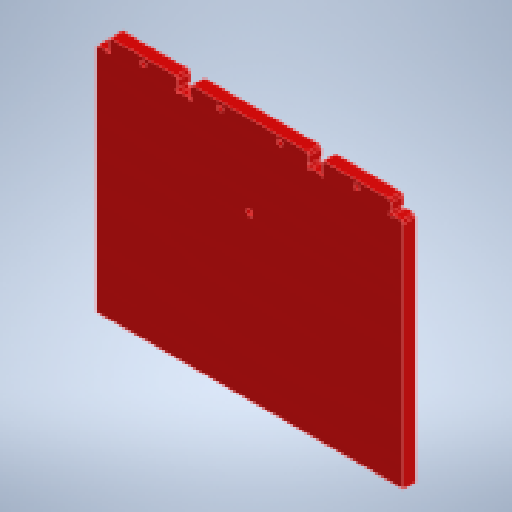
# Autodesk Inventor part: 부품49
Saved by Autodesk Inventor 2024 (Build 280153000, 153)
## iProperties
Created: 2024-09-07
Part Number: 부품49
Material: PMMA 플라스틱
Document SubType Name: Modeling
Designer: Eungang
Density: 1.188 g/cm^3
Appearance: 빨간색
Mass: 82.7023 g
Surface Area: 268.811 cm^2
Volume: 69.6147 cm^3
Author: Eungang
Autodesk Inventor part; units mm, degrees
ref_plane "YZ Plane" through (0, 0, 0) normal (1, 0, 0) x (0, 1, 0)
ref_plane "XZ Plane" through (0, 0, 0) normal (0, 1, 0) x (-1, 0, 0)
ref_plane "XY Plane" through (0, 0, 0) normal (0, 0, 1) x (1, 0, 0)
sketch "스케치1" plane through (0, 0, 0) normal (0, 0, 1) x (1, 0, 0)
  line L0 (118.1968, 6) -> (118.1968, 0)
  line L1 (0, 0) -> (2.3, 0) projected
  line L2 (2.3, 0) -> (2.3, -6) projected
  line L3 (150, -6) -> (2.3, -6) projected
  line L4 (150, -6) -> (150, 6) projected
  line L5 (0, 6) -> (150, 6) projected
  line L6 (0, 0) -> (0, 6) projected
  line L7 (150, -6) -> (0, -6)
  line L8 (0, -6) -> (0, 0)
  line L9 (0, 0) -> (150, 0)
  line L10 (150, 0) -> (150, -6)
  line L11 (150, -6) -> (144, -6)
  line L12 (144, -6) -> (144, 0)
  line L13 (144, 0) -> (150, 0)
  line L14 (150, 0) -> (150, -6)
  line L15 (122.25, 6) -> (131.75, 6) projected
  line L16 (128.025, 6) -> (128.025, 0)
  line L17 (125.975, 6) -> (125.975, 0)
  line L18 (127, 0) -> (127, 6)
  line L19 (104, 0) -> (104, -6)
  line L20 (104, -6) -> (110, -6)
  line L21 (110, -6) -> (110, 0)
  line L22 (110, 0) -> (104, 0)
  line L23 (104, 0) -> (104, -6)
  line L24 (75, -6) -> (75, 6)
  line L25 (0, 0) -> (0, -6)
  line L26 (0, -6) -> (6, -6)
  line L27 (6, 0) -> (0, 0)
  line L28 (0, 0) -> (0, -6)
  line L29 (40, 0) -> (46, 0)
  line L30 (150, -6) -> (144, -6)
  line L31 (144, -6) -> (144, 0)
  line L32 (144, 0) -> (150, 0)
  line L33 (150, 0) -> (150, -6)
  line L34 (110, -6) -> (104, -6)
  line L35 (104, -6) -> (104, 0)
  line L36 (104, 0) -> (110, 0)
  line L37 (110, 0) -> (110, -6)
  line L38 (0, 0) -> (0, -6)
  line L39 (0, -6) -> (6, -6)
  line L40 (6, -6) -> (6, 0)
  line L41 (6, 0) -> (0, 0)
  line L42 (0, 0) -> (0, -6)
  line L43 (40, -6) -> (40, 0)
  line L44 (46, -6) -> (40, -6)
  line L45 (46, 0) -> (46, -6)
  line L46 (46, 0) -> (46, -6)
  line L47 (40, 0) -> (46, 0)
  line L48 (0, -6) -> (6, -6)
  line L49 (6, -6) -> (6, 0)
  line L50 (6, 0) -> (0, 0)
  line L51 (0, 0) -> (0, -6)
  line L52 (40, -6) -> (46, -6)
  line L53 (46, -6) -> (46, 0)
  line L54 (46, 0) -> (40, 0)
  line L55 (40, 0) -> (40, -6)
  line L56 (150, 0) -> (0, 0)
  line L57 (0, 0) -> (0, -125.2)
  line L58 (0, -125.2) -> (150, -125.2)
  line L59 (150, -125.2) -> (150, 0)
  line L60 (150, -62.6) -> (0, -62.6)
  line L61 (0, -125.2) -> (2.3, -125.2)
  line L62 (2.3, -125.2) -> (2.3, -119.2)
  line L63 (150, -119.2) -> (2.3, -119.2)
  line L64 (150, -119.2) -> (0, -119.2)
  line L65 (0, -119.2) -> (0, -125.2)
  line L66 (0, -125.2) -> (150, -125.2)
  line L67 (150, -125.2) -> (150, -119.2)
  line L68 (150, -119.2) -> (144, -119.2)
  line L69 (144, -119.2) -> (144, -125.2)
  line L70 (144, -125.2) -> (150, -125.2)
  line L71 (150, -125.2) -> (150, -119.2)
  line L72 (110, -119.2) -> (110, -125.2)
  line L73 (104, -119.2) -> (110, -119.2)
  line L74 (104, -125.2) -> (104, -119.2)
  line L75 (104, -125.2) -> (104, -119.2)
  line L76 (110, -125.2) -> (104, -125.2)
  line L77 (40, -125.2) -> (46, -125.2)
  line L78 (0, -125.2) -> (0, -119.2)
  line L79 (0, -119.2) -> (6, -119.2)
  line L80 (0, -125.2) -> (0, -119.2)
  line L81 (6, -125.2) -> (0, -125.2)
  line L82 (150, -119.2) -> (144, -119.2)
  line L83 (144, -119.2) -> (144, -125.2)
  line L84 (144, -125.2) -> (150, -125.2)
  line L85 (150, -125.2) -> (150, -119.2)
  line L86 (110, -119.2) -> (104, -119.2)
  line L87 (104, -119.2) -> (104, -125.2)
  line L88 (104, -125.2) -> (110, -125.2)
  line L89 (110, -125.2) -> (110, -119.2)
  line L90 (0, -125.2) -> (0, -119.2)
  line L91 (0, -119.2) -> (6, -119.2)
  line L92 (6, -119.2) -> (6, -125.2)
  line L93 (6, -125.2) -> (0, -125.2)
  line L94 (0, -125.2) -> (0, -119.2)
  line L95 (6, -119.2) -> (6, -125.2)
  line L96 (0, -125.2) -> (0, -119.2)
  line L97 (0, -119.2) -> (6, -119.2)
  line L98 (6, -125.2) -> (0, -125.2)
  line L99 (40, -119.2) -> (40, -125.2)
  line L100 (40, -125.2) -> (40, -119.2)
  line L101 (46, -119.2) -> (40, -119.2)
  line L102 (46, -125.2) -> (46, -119.2)
  line L103 (46, -125.2) -> (46, -119.2)
  line L104 (46, -119.2) -> (46, -125.2)
  line L105 (40, -119.2) -> (46, -119.2)
  line L106 (46, -125.2) -> (40, -125.2)
  line L107 (40, -125.2) -> (46, -125.2)
  line L108 (150, -125.2) -> (0, -125.2)
  point P0 (21.975, 0)
  point P1 (24.025, 0)
  point P2 (31.8032, 0)
  point P3 (21.975, 0)
  point P4 (24.025, 0)
  point P5 (23, 0)
  point P6 (118.1968, -125.2)
  point P7 (128.025, -125.2)
  point P8 (125.975, -125.2)
  point P9 (127, -125.2)
  point P10 (75, -119.2)
  point P11 (24.025, -125.2)
  point P12 (21.975, -125.2)
  point P13 (24.025, -125.2)
  point P14 (23, -125.2)
  point P15 (21.975, -125.2)
  point P16 (31.8032, -125.2)
  dimension "d0" = 125.2
  constraints: 204 end point, 79 symmetric about line, 10 parallel, 5 horizontal, 5 midpoint, 5 perpendicular, 4 point on line, 3 vertical, 6 other
  measures "d0" distance of L57.end L56.end
extrude "돌출1" add sketch "스케치1" along normal blind 6 contours L9 L12 L3 L21 | L24 L3 L45 L9 | L9 L19 L3 L24 | L3 L59 L60 L57 L7 | L43 L3 L40 L9 | L60 L59 L63 L64 L57
sketch "스케치2" plane through (0, 0, 0) normal (0, 0, -1) x (-1, 0, 0)
  circle A0 centre (-72.2193, -29.1573) radius 1.55 projected
  circle A1 centre (-75, -39.8) radius 1.5 projected
  circle A2 centre (-75, -39.8) radius 13.9 projected
  circle A3 centre (-75, -39.8) radius 5.2 projected
  circle A4 centre (-75, -39.8) radius 1.6
  point P0 (0, 0)
  dimension "d5" = 0.1
  constraints: 1 centre point
  measures "d5" radial gap between concentric circles of A1 A4
extrude "돌출2" cut sketch "스케치2" against normal up to next contours A1 | A4
sketch "스케치5" plane through (0, 0, 6) normal (0, 0, 1) x (1, 0, 0)
  line L0 (6, 0) -> (6, -6) projected
  line L1 (6, -6) -> (0, -6) projected
  line L2 (0, -6) -> (0, -119.2) projected
  line L3 (150, -119.2) -> (150, -6) projected
  line L4 (150, -6) -> (144, -6) projected
  line L5 (144, -6) -> (144, 0) projected
  line L6 (144, 0) -> (110, 0) projected
  line L7 (110, 0) -> (110, -6) projected
  line L8 (110, -6) -> (104, -6) projected
  line L9 (104, -6) -> (104, 0) projected
  line L10 (104, 0) -> (46, 0) projected
  line L11 (46, 0) -> (46, -6) projected
  line L12 (46, -6) -> (40, -6) projected
  line L13 (40, -6) -> (40, 0) projected
  line L14 (40, 0) -> (6, 0) projected
  circle A0 centre (75, -39.8) radius 1.6 projected
  circle A1 centre (40, -6) radius 1
  circle A2 centre (46, -6) radius 1
  circle A3 centre (40, 0) radius 1
  circle A4 centre (46, 0) radius 1
  circle A5 centre (6, 0) radius 1
  line L15 (6, 0) -> (6, -6) projected
  circle A6 centre (6, -6) radius 1
  circle A7 centre (0, -6) radius 1
  circle A8 centre (104, -6) radius 1
  circle A9 centre (104, 0) radius 1
  line L16 (110, -6) -> (104, -6) projected
  circle A10 centre (110, -6) radius 1
  circle A11 centre (110, 0) radius 1
  circle A12 centre (144, -6) radius 1
  line L17 (144, 0) -> (110, 0) projected
  circle A13 centre (144, 0) radius 1
  circle A14 centre (150, -6) radius 1
  circle A15 centre (123.8, -69.5) radius 1
  circle A16 centre (123.8, -63.1) radius 1
  circle A17 centre (130.2, -69.5) radius 1
  line L18 (130.2, -69.5) -> (130.2, -63.1) projected
  circle A18 centre (130.2, -63.1) radius 1
  circle A19 centre (19.8, -69.5) radius 1
  circle A20 centre (19.8, -63.1) radius 1
  circle A21 centre (26.2, -69.5) radius 1
  circle A22 centre (26.2, -63.1) radius 1
  line L19 (0, -119.2) -> (150, -119.2) projected
  point P0 (0, 0)
  point P1 (149, -6)
  point P2 (150, -7)
  point P3 (144, -5)
  point P4 (145, -6)
  point P5 (143, 0)
  point P6 (144, -1)
  dimension "d32" = 2
  dimension "d33" = 2
  dimension "d34" = 2
  dimension "d35" = 2
  dimension "d36" = 2
  dimension "d37" = 2
  dimension "d38" = 2
  dimension "d39" = 2
  dimension "d40" = 2
  dimension "d41" = 2
  dimension "d42" = 2
  dimension "d43" = 2
  dimension "d44" = 2
  dimension "d45" = 2
  dimension "d46" = 2
  dimension "d47" = 2
  dimension "d48" = 2
  dimension "d49" = 2
  dimension "d50" = 2
  dimension "d51" = 2
  dimension "d52" = 2
  dimension "d53" = 2
  constraints: 22 centre point, 16 coincident
  measures "d32" diameter of A1
  measures "d33" diameter of A2
  measures "d34" diameter of A3
  measures "d35" diameter of A4
  measures "d36" diameter of A5
  measures "d37" diameter of A6
  measures "d38" diameter of A7
  measures "d39" diameter of A8
  measures "d40" diameter of A9
  measures "d41" diameter of A10
  measures "d42" diameter of A11
  measures "d43" diameter of A12
  measures "d44" diameter of A13
  measures "d45" diameter of A14
  measures "d46" diameter of A15
  measures "d47" diameter of A16
  measures "d48" diameter of A17
  measures "d49" diameter of A18
  measures "d50" diameter of A19
  measures "d51" diameter of A20
  measures "d52" diameter of A21
  measures "d53" diameter of A22
extrude "돌출5" cut sketch "스케치5" against normal up to next contours L14 A5 L0 | L0 A5 L14 | A6 L1 L0 | L0 L1 A6 | A3 L13 L14 | L14 L13 A3 | A7 L2 L1 | L1 L2 A7 | A1 L12 L13 | L13 L12 A1 | A2 L11 L12 | L12 L11 A2 | A14 L4 L3 | A4 L10 L11 | L11 L10 A4 | A12 L5 L4 | A9 L9 L10 | L10 L9 A9 | A13 L6 L5 | A8 L8 L9 | L9 L8 A8 | A11 L7 L6 | L6 L7 A11 | A10 L7 L8 | L8 L7 A10 picked at (149.7812, -6.6253) picked at (143.8112, -6.634) picked at (143.7812, -0.6253)
sketch "스케치6" plane through (0, 0, 6) normal (0, 0, 1) x (1, 0, 0)
  line L0 (6, -6) -> (6, 0) projected
  line L1 (0, 0) -> (6, 0) projected
  line L2 (0, -6) -> (0, 0) projected
  line L3 (0, -6) -> (6, -6) projected
  line L4 (40, 0) -> (40, -6) projected
  line L5 (40, -6) -> (46, -6) projected
  line L6 (46, -6) -> (46, 0) projected
  line L7 (40, 0) -> (46, 0) projected
  line L8 (40, 0) -> (6, 0)
  line L9 (23, 0) -> (23, -6)
  circle A0 centre (23, -3) radius 1.35
  line L10 (104, 0) -> (104, -6) projected
  line L11 (104, -6) -> (110, -6) projected
  line L12 (110, -6) -> (110, 0) projected
  line L13 (104, 0) -> (110, 0) projected
  line L14 (144, 0) -> (144, -6) projected
  line L15 (144, -6) -> (150, -6) projected
  line L16 (150, -6) -> (150, 0) projected
  line L17 (144, 0) -> (150, 0) projected
  line L18 (104, -3) -> (46, -3)
  line L19 (75, -3) -> (75, 0)
  line L20 (103, 0) -> (47, 0) projected
  line L21 (75, -3) -> (104, -3)
  line L22 (89.5, -3) -> (89.5, 0)
  line L23 (75, -3) -> (46, -3)
  line L24 (60.5, -3) -> (60.5, 0)
  circle A1 centre (89.5, -3) radius 1.3
  circle A2 centre (60.5, -3) radius 1.3
  circle A3 centre (127, -3) radius 1.35
  point P0 (127, -6)
  dimension "d58" = 2.6
  dimension "d59" = 2.6
  constraints: 16 end point, 8 midpoint, 4 centre point, 2 coincident, 2 collinear, 2 perpendicular, 2 symmetric about line, 2 vertical, 1 point on line, 1 other
  measures "d58" diameter of A1
  measures "d59" diameter of A2
extrude "돌출6" cut sketch "스케치6" against normal up to next contours A0 L9 | L9 A0 | A1 L18 | L18 L22 A1 | L18 A1 L22 | A2 L18 | L18 L24 A2 | L18 A2 L24 | A3
sketch "스케치13" plane through (0, 0, 6) normal (0, 0, 1) x (1, 0, 0)
  circle A0 centre (82.7782, -32.0218) radius 1.55 projected
  circle A1 centre (82.7782, -32.0218) radius 1.55 projected
  circle A2 centre (75, -28.8) radius 1.55 projected
  circle A3 centre (75, -39.8) radius 1.6 projected
  circle A4 centre (82.7782, -32.0218) radius 1.55
  circle A5 centre (75, -28.8) radius 1.55
  circle A6 centre (67.2218, -32.0218) radius 1.55
  circle A7 centre (64, -39.8) radius 1.55
  circle A8 centre (67.2218, -47.5782) radius 1.55
  circle A9 centre (75, -50.8) radius 1.55
  circle A10 centre (82.7782, -47.5782) radius 1.55
  circle A11 centre (86, -39.8) radius 1.55
  point P0 (0, 0)
  dimension "d77" = 360
  constraints: 8 centre point, 1 coincident, 1 concentric, 17 other
extrude "돌출9" cut sketch "스케치13" against normal blind 10 contours A0 | A2 | A6 | A7 | A8 | A9 | A10 | A11
